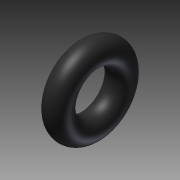
# Autodesk Inventor part: 9452K14 Buna-N O-Ring
Saved by Autodesk Inventor 2012 SP1 (Build 160190100, 190)
## iProperties
Created: 2012-06-04
Part Number: 9452K14 Buna-N O-Ring
Material: Rubber
Document SubType Name: Modeling
Designer: ding42
Mass: 0.0337749 g
Surface Area: 0.818164 cm^2
Volume: 0.0363171 cm^3
Density: 0.93 g/cm^3
Description: Dash Number 006
Author: ding42
Autodesk Inventor part; units mm, degrees
ref_plane "YZ Plane" through (0, 0, 0) normal (1, 0, 0) x (0, 1, 0)
ref_plane "XZ Plane" through (0, 0, 0) normal (0, 1, 0) x (-1, 0, 0)
ref_plane "XY Plane" through (0, 0, 0) normal (0, 0, 1) x (1, 0, 0)
sketch "Sketch1" plane through (0, 0, 0) normal (0, 0, 1) x (1, 0, 0)
  circle A0 centre (0, 0) radius 0.889
  dimension "d0" = 1.778
  constraints: 1 centre point, 1 coincident
  measures "d0" diameter of A0
sketch "Sketch2" plane through (0, 0, 0) normal (1, 0, 0) x (0, 1, 0)
  circle A0 centre (2.328, -0.1597) radius 1.4478
  line L0 (0.889, 0) -> (-0.889, 0) projected
  point P0 (0, 0)
  dimension "d1" = 2.8956
  constraints: 3 other
sweep "Sweep1" add profiles "Sketch1" path "Sketch2" path curves A0
body "Solid1"
